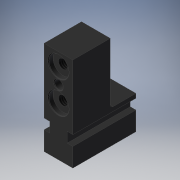
# Autodesk Inventor part: 1254044 DHPS-16-A-NO---(Handle)
Saved by Autodesk Inventor 2019 (Build 230136000, 136)
## iProperties
Created: 2023-01-29
Part Number: 1254044 DHPS-16-A-NO---(Handle)
Material: Generic
Catalog Web Link: www.cadenas.de
Description: DHPS---(Handle)-Handle
Vendor: FESTO
Document SubType Name: Modeling
Designer: psAdmin
Manufacturer: FESTO
Mass: 4.5385 g
Surface Area: 26.6044 cm^2
Volume: 4.5385 cm^3
Density: 1 g/cm^3
Appearance: PSOLRGB-175-175-175
Category: PARTsolutions
Company: FESTO
Title: 1254044 DHPS-16-A-NO---(Handle)
Author: Cadenas PARTsolutions
Comments: Handle
PSOL_IDENT_0: {$CADENAS_DATA/23d-libs/festo/parts/d/dhps/parts/dhps_griff.prj},211 {VTYP=3D},{NB=1254044 DHPS-16-A
PSOL_IDENT_1: -NO---(Handle)},{LINA=1254044 DHPS-16-A-NO---(Handle)},{NN=DHPS---(Handle)},{DATE=03.06.2022 12:54:4
PSOL_IDENT_2: 1},{GEOMDATE=03.06.2022 11:49:00},{VERSION=},{LINEID=60},{WBVAR=},{WBNUMERIC=}  {NB=1254044 DHPS-16-
PSOL_IDENT_3: A-NO---(Griff)},{LINA=1254044 DHPS-16-A-NO---(Griff)},{KT=DUMMY},{TNR=1254044},{TYP=DHPS-16-A-NO},{G
PSOL_IDENT_4: R=16},{B1=10.000},{B2=6.000},{H1=32.500},{H2=6.500},{H3=3.550},{H4=11.500},{H5=17.000},{H6=11.000},{
PSOL_IDENT_5: H7=22.500},{L1=21.900},{L2=8.900},{L3=1.600},{D1=3.400},{D2=3.000},{D3=4.000},{D4=7.000},{R1=1.000},
PSOL_IDENT_6: {HCL=1.500},{HCH=1.500},{HCW=1.500},{HCX=1.500},{VERS=6}
NB: 1254044 DHPS-16-A-NO---(Handle)
NN: DHPS---(Handle)
NT: Handle
NBSYN: $TNR. $TYP.---(Handle)
LINA: 1254044 DHPS-16-A-NO---(Handle)
CATALOG: Festo
TNR: 1254044
TYP: DHPS-16-A-NO
GR: 16
B1: 10
B2: 6
H1: 32.5
H2: 6.5
H3: 3.55
H4: 11.5
H5: 17
H6: 11
H7: 22.5
L1: 21.9
L2: 8.9
L3: 1.6
D1: 3.4
D2: 3
D3: 4
D4: 7
R1: 1
HCL: 1.5
HCH: 1.5
HCW: 1.5
HCX: 1.5
VERS: 6
SUPPLIER: FESTO
ARTICLENO: 1254044 DHPS-16-A-NO---(Handle)
BOMINFO: 1254044 DHPS-16-A-NO---(Handle)
CREATOR: CADENAS GmbH
Autodesk Inventor part; units mm, degrees
ref_plane "YZ Plane" through (0, 0, 0) normal (1, 0, 0) x (0, 1, 0)
ref_plane "XZ Plane" through (0, 0, 0) normal (0, 1, 0) x (-1, 0, 0)
ref_plane "XY Plane" through (0, 0, 0) normal (0, 0, 1) x (1, 0, 0)
sketch "Sketch_1" plane through (0, 0, 0) normal (0, 0, 1) x (1, 0, 0)
  line L0 (-5, 10.05) -> (-3, 10.05)
  line L1 (-3, 10.05) -> (-3, 6.5)
  line L2 (-3, 6.5) -> (-5, 6.5)
  line L3 (-5, 6.5) -> (-5, 0)
  line L4 (-5, 0) -> (5, 0)
  line L5 (5, 0) -> (5, 6.5)
  line L6 (5, 6.5) -> (3, 6.5)
  line L7 (3, 6.5) -> (3, 10.05)
  line L8 (3, 10.05) -> (5, 10.05)
  line L9 (5, 10.05) -> (5, 32.5)
  line L10 (5, 32.5) -> (-5, 32.5)
  line L11 (-5, 32.5) -> (-5, 10.05)
  constraints: 24 end point
extrude "Extrusion1" add sketch "Sketch_1" along normal blind 21.9
sketch "Sketch_2" plane through (0, 0, 0) normal (1, 0, 0) x (0, 1, 0)
  arc A0 (12.5, 8.9) -> (11.5, 7.9) centre (12.5, 7.9) ccw
  line L0 (11.5, 7.9) -> (11.5, 0)
  line L1 (11.5, 0) -> (32.5, 0)
  line L2 (32.5, 0) -> (32.5, 8.9)
  line L3 (32.5, 8.9) -> (12.5, 8.9)
  constraints: 8 end point, 2 point on circle, 1 centre point
extrude "Extrusion2" cut sketch "Sketch_2" along normal mid plane 10
sketch "Sketch_5" plane through (0, 0, 0) normal (1, 0, 0) x (0, 1, 0)
  line L0 (22.5, 8.9) -> (22.5, 21.9)
  line L1 (22.5, 21.9) -> (24.2, 21.9)
  line L2 (24.2, 21.9) -> (24, 21.7)
  line L3 (24, 21.7) -> (24, 9.1)
  line L4 (24, 9.1) -> (24.2, 8.9)
  line L5 (24.2, 8.9) -> (22.5, 8.9)
  line L6 (22.5, 8.9) -> (22.5, 21.9)
  constraints: 14 end point
revolve "Revolution1" cut sketch "Sketch_5" angle 360 about axis through (0, 22.5, 8.9) along (0, 0, -1)
sketch "Sketch_6" plane through (0, 0, 0) normal (1, 0, 0) x (0, 1, 0)
  line L0 (17, 8.9) -> (17, 21.9)
  line L1 (17, 21.9) -> (20.7, 21.9)
  line L2 (20.7, 21.9) -> (20.5, 21.7)
  line L3 (20.5, 21.7) -> (20.5, 20.3)
  line L4 (20.5, 20.3) -> (18.621, 20.3)
  line L5 (18.621, 20.3) -> (18.621, 8.9)
  line L6 (18.621, 8.9) -> (17, 8.9)
  line L7 (17, 8.9) -> (17, 21.9)
  constraints: 16 end point
revolve "Revolution2" cut sketch "Sketch_6" angle 360 about axis through (0, 17, 8.9) along (0, 0, -1)
thread "Thread1" size "M4x0.7" class "6H" standard "ISO Metric profile" full length
sketch "Sketch_7" plane through (0, 0, 0) normal (1, 0, 0) x (0, 1, 0)
  line L0 (28, 8.9) -> (28, 21.9)
  line L1 (28, 21.9) -> (31.7, 21.9)
  line L2 (31.7, 21.9) -> (31.5, 21.7)
  line L3 (31.5, 21.7) -> (31.5, 20.3)
  line L4 (31.5, 20.3) -> (29.621, 20.3)
  line L5 (29.621, 20.3) -> (29.621, 8.9)
  line L6 (29.621, 8.9) -> (28, 8.9)
  line L7 (28, 8.9) -> (28, 21.9)
  constraints: 16 end point
revolve "Revolution3" cut sketch "Sketch_7" angle 360 about axis through (0, 28, 8.9) along (0, 0, -1)
thread "Thread2" size "M4x0.7" class "6H" standard "ISO Metric profile" full length
sketch "Sketch_10" plane through (0, 0, 0) normal (0, 1, 0) x (-1, 0, 0)
  line L0 (0.75, 3) -> (-0.75, 3)
  line L1 (-0.75, 3) -> (-0.75, 1.5)
  line L2 (-0.75, 1.5) -> (0.75, 1.5)
  line L3 (0.75, 1.5) -> (0.75, 3)
  constraints: 8 end point
extrude "Extrusion3" add sketch "Sketch_10" against normal blind 1.5
ref_plane "GRIFF_XY" through (0, 0, 0) normal (0, 0, -1) x (1, 0, 0)
ref_plane "GRIFF_YZ" through (0, 0, 0) normal (1, 0, 0) x (0, -1, 0)
ref_plane "GRIFF_ZX" through (0, 0, 0) normal (0, -1, 0) x (0, 0, -1)
ref_plane "TO_ZBH_1_XY" through (0, 17, 20.3) normal (0, 0, -1) x (1, 0, 0)
ref_plane "TO_ZBH_1_YZ" through (0, 17, 20.3) normal (1, 0, 0) x (0, -1, 0)
ref_plane "TO_ZBH_1_ZX" through (0, 17, 20.3) normal (0, -1, 0) x (0, 0, -1)
ref_plane "TO_ZBH_2_XY" through (0, 28, 20.3) normal (0, 0, -1) x (1, 0, 0)
ref_plane "TO_ZBH_2_YZ" through (0, 28, 20.3) normal (1, 0, 0) x (0, -1, 0)
ref_plane "TO_ZBH_2_ZX" through (0, 28, 20.3) normal (0, -1, 0) x (0, 0, -1)
body "Solid1"
